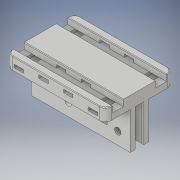
# Autodesk Inventor part: RadioPanelMountA
Saved by Autodesk Inventor 2018 (Build 220112000, 112)
## iProperties
Created: 2017-09-07
Part Number: RadioPanelMountA
Material: Generic
Document SubType Name: Modeling
Designer: Srinity
Density: 1 g/cm^3
Appearance: Default
Author: Srinity
Autodesk Inventor part; units mm, degrees
ref_plane "YZ Plane" through (0, 0, 0) normal (1, 0, 0) x (0, 1, 0)
ref_plane "XZ Plane" through (0, 0, 0) normal (0, 1, 0) x (-1, 0, 0)
sketch "Sketch1" plane through (0, 0, 0) normal (1, 0, 0) x (0, 1, 0)
  line L0 (31.75, 34.925) -> (19.05, 34.925)
  line L1 (19.05, 34.925) -> (19.05, 9.525)
  line L2 (19.05, -34.925) -> (31.75, -34.925)
  line L3 (31.75, -34.925) -> (31.75, 34.925)
  line L4 (19.05, 9.525) -> (-19.05, 9.525)
  line L5 (-19.05, 9.525) -> (-19.05, 3.175)
  line L6 (-19.05, 3.175) -> (19.05, 3.175)
  line L7 (19.05, 3.175) -> (19.05, 9.525) construction
  line L8 (19.05, -3.175) -> (-19.05, -3.175)
  line L9 (-19.05, -3.175) -> (-19.05, -9.525)
  line L10 (-19.05, -9.525) -> (19.05, -9.525)
  line L11 (19.05, -9.525) -> (19.05, -3.175) construction
  line L12 (19.05, 3.175) -> (19.05, -3.175)
  line L13 (19.05, -9.525) -> (19.05, -34.925)
  point P0 (0, 0)
  dimension "d0" = 12.7
  dimension "d1" = 6.35
  dimension "d2" = 38.1
  dimension "d3" = 6.35
  dimension "d4" = 19.05
  dimension "d5" = 3.175
  dimension "d6" = 69.85
  dimension "d7" = 19.05
  dimension "d8" = 25.4
  constraints: 28 end point, 8 parallel, 5 perpendicular, 3 horizontal, 2 collinear, 1 point on line
  measures "d0" distance of L0.start L0.end
  measures "d1" distance between parallel lines of L8 L6
  measures "d2" distance of L1.end L4.end
  measures "d3" distance of L4.end L5.end
  measures "d4" distance from line of L12 point (0, 0)
  measures "d5" distance from line of L8 point (0, 0)
  measures "d6" distance of L2.end L0.start
  measures "d7" distance between parallel lines of L10 L4
  measures "d8" distance of L0.end L1.end
extrude "Extrusion1" add sketch "Sketch1" along normal blind 101.6
sketch "Sketch2" plane through (0, 19.05, -34.925) normal (0, -1, 0) x (1, 0, 0)
  line L0 (0, 0) -> (101.6, 0) projected
  line L1 (23.8125, 25.4) -> (26.9875, 25.4)
  line L2 (26.9875, 25.4) -> (26.9875, 0)
  line L3 (26.9875, 0) -> (23.8125, 0)
  line L4 (23.8125, 0) -> (23.8125, 25.4)
  line L5 (0, 25.4) -> (101.6, 25.4) projected
  line L6 (0, 25.4) -> (0, 0) projected
  line L7 (49.2125, 25.4) -> (52.3875, 25.4)
  line L8 (52.3875, 25.4) -> (52.3875, 0)
  line L9 (52.3875, 0) -> (49.2125, 0)
  line L10 (49.2125, 0) -> (49.2125, 25.4)
  line L11 (74.6125, 25.4) -> (77.7875, 25.4)
  line L12 (77.7875, 25.4) -> (77.7875, 0)
  line L13 (77.7875, 0) -> (74.6125, 0)
  line L14 (74.6125, 0) -> (74.6125, 25.4)
  point P0 (0, 34.925)
  dimension "d11" = 3.175
  dimension "d12" = 23.8125
  dimension "d15" = 25.4
  constraints: 24 end point, 2 horizontal, 2 parallel, 1 collinear, 1 perpendicular, 1 point on line, 16 other
  measures "d11" distance between parallel lines of L2 L4
  measures "d12" distance between parallel lines of L4 L6
  measures "d15" distance of L1.start L7.start
extrude "Extrusion2" add sketch "Sketch2" along normal blind 25.4 contours L4 L1 L2 L0 | L10 L5 L8 L0 | L14 L5 L12 L0
chamfer "Chamfer1" distance 25.4 angle 45 3 edges at (25.4, -6.35, -34.925) (50.8, -6.35, -34.925) (76.2, -6.35, -34.925)
ref_plane "Work Plane1" through (0, -19.05, 0) normal (0, 0, -1) x (-1, 0, 0)
mirror "Mirror1" about plane through (0, -19.05, 0) normal (0, 0, -1) of "Extrusion2", "Chamfer1"
fillet "Fillet1" radius 6.35 4 edges at (0, 25.4, -34.925) (101.6, 25.4, -34.925) (101.6, 25.4, 34.925) (0, 25.4, 34.925)
chamfer "Chamfer2" distance 1.27 angle 45 2 edges at (50.8, -19.05, -3.175) (50.8, -19.05, 3.175)
sketch "Sketch3" plane through (26.9875, 19.05, 34.925) normal (0, 0, 1) x (1, 0, 0)
  line L0 (66.675, 3.175) -> (57.15, 3.175)
  line L1 (57.15, 3.175) -> (57.15, 6.35)
  line L2 (57.15, 6.35) -> (66.675, 6.35)
  line L3 (66.675, 6.35) -> (66.675, 3.175)
  line L4 (41.275, 6.35) -> (31.75, 6.35)
  line L5 (31.75, 6.35) -> (31.75, 9.525)
  line L6 (31.75, 9.525) -> (41.275, 9.525)
  line L7 (41.275, 9.525) -> (41.275, 6.35)
  line L8 (15.875, 6.35) -> (6.35, 6.35)
  line L9 (6.35, 6.35) -> (6.35, 9.525)
  line L10 (6.35, 9.525) -> (15.875, 9.525)
  line L11 (15.875, 9.525) -> (15.875, 6.35)
  line L12 (-9.525, 3.175) -> (-19.05, 3.175)
  line L13 (-19.05, 3.175) -> (-19.05, 6.35)
  line L14 (-19.05, 6.35) -> (-9.525, 6.35)
  line L15 (-9.525, 6.35) -> (-9.525, 3.175)
  line L16 (-20.6375, 12.7) -> (68.2625, 12.7) projected
  line L17 (61.9125, 3.175) -> (61.9125, 6.35) construction
  line L18 (74.6125, 0) -> (74.6125, -38.1) projected
  line L19 (36.5125, 6.35) -> (36.5125, 9.525) construction
  line L20 (11.1125, 6.35) -> (11.1125, 9.525) construction
  line L21 (-14.2875, 3.175) -> (-14.2875, 6.35) construction
  point P0 (-26.9875, -19.05)
  dimension "d29" = 9.525
  dimension "d30" = 3.175
  dimension "d31" = 6.35
  dimension "d32" = 12.7
  dimension "d33" = 25.4
  dimension "d34" = 25.4
  dimension "d35" = 25.4
  dimension "d63" = 3.175
  dimension "d64" = 3.175
  constraints: 40 end point, 8 midpoint, 8 parallel, 4 perpendicular, 3 equal length, 3 horizontal, 2 collinear, 2 point on line
  measures "d29" distance of L0.start L0.end
  measures "d30" distance of L0.end L1.end
  measures "d31" distance between parallel lines of L2 L16
  measures "d32" distance between parallel lines of L17 L18
  measures "d33" distance between parallel lines of L19 L17
  measures "d34" distance between parallel lines of L20 L19
  measures "d35" distance between parallel lines of L21 L20
  measures "d63" distance between parallel lines of L6 L16
  measures "d64" distance of L6.end L4.start
extrude "Extrusion3" cut sketch "Sketch3" against normal through all
sketch "Sketch4" plane through (101.6, 0, 0) normal (1, 0, 0) x (0, 0, -1)
  line L0 (28.575, 31.75) -> (-28.575, 31.75) projected
  line L1 (-27.6225, 31.75) -> (-16.8275, 31.75)
  line L2 (-16.8275, 31.75) -> (-16.8275, 25.4)
  line L3 (-16.8275, 25.4) -> (-27.6225, 25.4)
  line L4 (-27.6225, 25.4) -> (-27.6225, 31.75)
  line L5 (16.8275, 31.75) -> (27.6225, 31.75)
  line L6 (27.6225, 31.75) -> (27.6225, 25.4)
  line L7 (27.6225, 25.4) -> (16.8275, 25.4)
  line L8 (16.8275, 25.4) -> (16.8275, 31.75)
  line L9 (-22.225, 31.75) -> (-22.225, 25.4) construction
  line L10 (22.225, 31.75) -> (22.225, 25.4) construction
  line L11 (-34.925, 25.4) -> (34.925, 25.4) projected
  line L12 (-34.925, 31.75) -> (-34.925, 19.05) projected
  line L13 (34.925, 19.05) -> (34.925, 31.75) projected
  point P0 (0, 0)
  dimension "d38" = 10.795
  dimension "d39" = 6.35
  dimension "d40" = 12.7
  dimension "d41" = 12.7
  constraints: 20 end point, 4 parallel, 4 point on line, 3 midpoint, 3 perpendicular, 2 horizontal, 1 collinear
  measures "d38" distance of L2.end L3.end
  measures "d39" distance of L1.end L2.end
  measures "d40" distance between parallel lines of L12 L9
  measures "d41" distance between parallel lines of L10 L13
extrude "Extrusion4" cut sketch "Sketch4" against normal through all contours L6 L7 L8 L0 | L2 L3 L4 L0
chamfer "Chamfer3" distance 0.635 angle 45 10 edges at (50.8, 31.75, 34.925) (99.7401, 31.75, 33.0651) (1.8599, 31.75, 33.0651) (50.8, 31.75, 27.6225) (50.8, 31.75, 16.8275) (50.8, 31.75, -16.8275) (50.8, 31.75, -27.6225) (50.8, 31.75, -34.925) (99.7401, 31.75, -33.0651) (1.8599, 31.75, -33.0651)
sketch "Sketch5" plane through (7.9375, 22.225, 34.925) normal (0, 1, 0) x (1, 0, 0)
  line L0 (16.1925, 62.5475) -> (69.5325, 62.5475)
  line L1 (69.5325, 62.5475) -> (69.5325, 51.7525)
  line L2 (69.5325, 51.7525) -> (16.1925, 51.7525)
  line L3 (16.1925, 51.7525) -> (16.1925, 62.5475)
  line L4 (16.1925, 18.0975) -> (69.5325, 18.0975)
  line L5 (69.5325, 18.0975) -> (69.5325, 7.3025)
  line L6 (69.5325, 7.3025) -> (16.1925, 7.3025)
  line L7 (16.1925, 7.3025) -> (16.1925, 18.0975)
  line L8 (-7.9375, 62.5475) -> (93.6625, 62.5475) projected
  line L9 (93.6625, 51.7525) -> (-7.9375, 51.7525) projected
  line L10 (-7.9375, 18.0975) -> (93.6625, 18.0975) projected
  line L11 (-7.9375, 51.7525) -> (-7.9375, 62.5475) projected
  point P0 (-7.9375, 34.925)
  point P1 (-7.9362, 63.627)
  point P2 (93.6612, 63.627)
  point P3 (-7.9375, 63.5)
  point P4 (93.6625, 62.5475)
  dimension "d47" = 53.34
  dimension "d48" = 24.13
  constraints: 16 end point, 4 parallel, 3 collinear, 3 horizontal, 2 equal length, 2 perpendicular, 1 other
  measures "d47" distance between parallel lines of L1 L3
  measures "d48" distance between parallel lines of L3 L11
extrude "Extrusion5" cut sketch "Sketch5" against normal blind 3.175 contours L0 L1 L2 L3 | L4 L5 L6 L7
sketch "Sketch6" plane through (0, -19.05, 9.525) normal (0, 0, 1) x (1, 0, 0)
  circle A0 centre (12.7, 25.4) radius 3.302
  circle A1 centre (38.1, 12.7) radius 3.302
  circle A2 centre (63.5, 25.4) radius 3.302
  circle A3 centre (88.9, 12.7) radius 3.302
  line L0 (0, 0) -> (101.6, 0) projected
  line L1 (0, 38.1) -> (0, 0) projected
  point P0 (0, 19.05)
  dimension "d51" = 12.7
  dimension "d52" = 12.7
  dimension "d53" = 6.604
  dimension "d54" = 12.7
  dimension "d55" = 25.4
  dimension "d56" = 25.4
  dimension "d57" = 25.4
  constraints: 4 centre point, 3 equal radius, 2 horizontal alignment
  measures "d51" vertical distance of A1.centre A0.centre
  measures "d52" distance from line of L0 A1.centre
  measures "d53" diameter of A0
  measures "d54" distance from line of A0.centre L1
  measures "d55" horizontal distance of A1.centre A0.centre
  measures "d56" horizontal distance of A2.centre A1.centre
  measures "d57" horizontal distance of A2.centre A3.centre
extrude "Extrusion6" cut sketch "Sketch6" against normal through all
chamfer "Chamfer4" distance 1.27 angle 45 4 edges at (0, 0.635, -3.175) (0, 0.635, 3.175) (101.6, 0.635, 3.175) (101.6, 0.635, -3.175)
equation "\"d4\" = 0.5 * d2"
equation "\"d5\" = 0.5 * d1"
equation "\"d8\" = -0.5 * d7 + 0.5 * d6"
body "Solid1"
